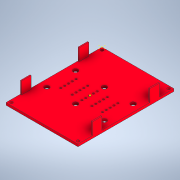
# Autodesk Inventor part: Base
Saved by Autodesk Inventor 2021 (Build 250183000, 183)
## iProperties
Created: 2025-01-23
Part Number: Base
Material: Generic
Document SubType Name: Modeling
Designer: User
Density: 1 g/cm^3
Appearance: Default
Author: User
Autodesk Inventor part; units mm, degrees
ref_plane "YZ Plane" through (0, 0, 0) normal (1, 0, 0) x (0, 1, 0)
ref_plane "XZ Plane" through (0, 0, 0) normal (0, 1, 0) x (-1, 0, 0)
ref_plane "XY Plane" through (0, 0, 0) normal (0, 0, 1) x (1, 0, 0)
sketch "Sketch1" plane through (0, 0, 0) normal (0, 1, 0) x (-1, 0, 0)
  line L0 (75, 0) -> (75, -100)
  line L1 (75, -100) -> (-75, -100)
  line L2 (-75, -100) -> (-75, 100)
  line L3 (-75, 100) -> (75, 100)
  line L4 (75, 100) -> (75, 0)
  line L5 (75, 100) -> (75, 70)
  line L6 (75, -100) -> (75, -70)
  line L7 (-75, -100) -> (-75, -70)
  line L8 (-75, 100) -> (-75, 70)
  line L9 (75, 70) -> (75, 50)
  line L10 (-75, 70) -> (-75, 50)
  line L11 (-75, -70) -> (-75, -50)
  line L12 (75, -70) -> (75, -50)
  line L13 (75, -70) -> (72.5, -70)
  line L14 (72.5, -70) -> (72.5, -50)
  line L15 (72.5, -50) -> (75, -50)
  line L16 (-75, -70) -> (-72.5, -70)
  line L17 (-72.5, -70) -> (-72.5, -50)
  line L18 (-72.5, -50) -> (-75, -50)
  line L19 (75, 70) -> (72.5, 70)
  line L20 (72.5, 70) -> (72.5, 50)
  line L21 (72.5, 50) -> (75, 50)
  line L22 (-75, 70) -> (-72.5, 70)
  line L23 (-72.5, 70) -> (-72.5, 50)
  line L24 (-72.5, 50) -> (-75, 50)
  line L25 (-75, -100) -> (-75, -97)
  line L26 (-75, -100) -> (-72, -100)
  circle A0 centre (-69.4679, -94.4422) radius 3
  circle A1 centre (69.3699, -94.4422) radius 3
  circle A2 centre (69.3699, 94.4217) radius 3
  circle A3 centre (-69.4679, 94.4217) radius 3
  line L27 (75, -50) -> (75, -35)
  line L28 (75, 50) -> (75, 35)
  line L29 (75, -35) -> (75, -25)
  line L30 (75, 35) -> (75, 25)
  line L31 (75, -25) -> (75, -21)
  line L32 (75, -21) -> (75, -17)
  line L33 (75, -17) -> (75, -13)
  line L34 (75, -13) -> (75, -9)
  line L35 (75, -9) -> (75, -5)
  line L36 (75, -5) -> (75, -1)
  line L37 (75, -1) -> (75, 3)
  line L38 (75, 3) -> (75, 7)
  line L39 (75, 7) -> (75, 11)
  line L40 (75, 11) -> (75, 15)
  line L41 (75, 15) -> (75, 19)
  line L42 (75, 19) -> (75, 23)
  circle A4 centre (60, 30) radius 5
  circle A5 centre (-60, 30) radius 5
  circle A6 centre (0, 30) radius 5
  line L43 (0, -35) -> (0, -30)
  circle A7 centre (0, -30) radius 5
  circle A8 centre (-60, -30) radius 5
  circle A9 centre (60, -30) radius 5
  circle A10 centre (0, -15) radius 2
  circle A11 centre (20, -15) radius 2
  circle A12 centre (44, -15) radius 2
  circle A13 centre (-21, -15) radius 2
  circle A14 centre (-43, -15) radius 2
  circle A15 centre (44, -7) radius 2
  circle A16 centre (20, -7) radius 2
  circle A17 centre (0, -7) radius 2
  circle A18 centre (-21, -7) radius 2
  circle A19 centre (-43, -7) radius 2
  circle A20 centre (44, 1) radius 2
  circle A21 centre (20, 1) radius 2
  circle A22 centre (0, 1) radius 2
  circle A23 centre (-21, 1) radius 2
  circle A24 centre (-43, 1) radius 2
  circle A25 centre (44, 9) radius 2
  circle A26 centre (20, 9) radius 2
  circle A27 centre (0, 9) radius 2
  circle A28 centre (-21, 9) radius 2
  circle A29 centre (-43, 9) radius 2
  circle A30 centre (44, 17) radius 2
  circle A31 centre (20, 17) radius 2
  circle A32 centre (0, 17) radius 2
  circle A33 centre (-21, 17) radius 2
  circle A34 centre (-43, 17) radius 2
  point P0 (0, 0)
  dimension "d3" = 150
  dimension "d4" = 200
  dimension "d6" = 30
  dimension "d7" = 30
  dimension "d8" = 30
  dimension "d9" = 30
  dimension "d10" = 20
  dimension "d11" = 20
  dimension "d12" = 20
  dimension "d13" = 20
  dimension "d14" = 2.5
  dimension "d15" = 2.5
  dimension "d16" = 2.5
  dimension "d17" = 2.5
  dimension "d20" = 6
  dimension "d23" = 6
  dimension "d26" = 6
  dimension "d28" = 6
  dimension "d30" = 15
  dimension "d31" = 15
  dimension "d32" = 10
  dimension "d33" = 10
  dimension "d34" = 4
  dimension "d35" = 4
  dimension "d47" = 10
  dimension "d49" = 10
  dimension "d50" = 10
  dimension "d51" = 5
  dimension "d52" = 10
  dimension "d55" = 10
  dimension "d56" = 10
  dimension "d58" = 4
  dimension "d59" = 4
  dimension "d60" = 4
  dimension "d61" = 4
  dimension "d62" = 4
  dimension "d63" = 4
  dimension "d64" = 4
  dimension "d65" = 4
  dimension "d66" = 4
  dimension "d67" = 4
  dimension "d68" = 4
  dimension "d69" = 4
  dimension "d70" = 4
  dimension "d71" = 4
  dimension "d72" = 4
  dimension "d73" = 4
  dimension "d74" = 4
  dimension "d75" = 4
  dimension "d76" = 4
  dimension "d77" = 4
  dimension "d78" = 4
  dimension "d79" = 4
  dimension "d80" = 4
  dimension "d81" = 4
  dimension "d82" = 4
  constraints: 84 end point, 35 centre point, 10 perpendicular, 6 point on line, 4 horizontal, 1 coincident, 1 vertical, 27 other
  measures "d3" distance of L1.start L1.end
  measures "d4" distance of L1.end L2.end
  measures "d6" distance of L3.end L5.end
  measures "d7" distance of L1.start L6.end
  measures "d8" distance of L1.end L7.end
  measures "d9" distance of L2.end L8.end
  measures "d10" distance of L5.end L9.end
  measures "d11" distance of L8.end L10.end
  measures "d12" distance of L7.end L11.end
  measures "d13" distance of L6.end L12.end
  measures "d14" distance of L6.end L13.end
  measures "d15" distance of L7.end L16.end
  measures "d16" distance of L5.end L19.end
  measures "d17" distance of L8.end L22.end
  measures "d20" diameter of A0
  measures "d23" diameter of A1
  measures "d26" diameter of A2
  measures "d28" diameter of A3
  measures "d30" distance of L12.end L27.end
  measures "d31" distance of L9.end L28.end
  measures "d32" distance of L27.end L29.end
  measures "d33" distance of L28.end L30.end
  measures "d34" distance of L29.end L31.end
  measures "d35" distance of L31.end L32.end
  measures "d47" diameter of A4
  measures "d49" diameter of A5
  measures "d50" diameter of A6
  measures "d51" distance of L43.start L43.end
  measures "d52" diameter of A7
  measures "d55" diameter of A8
  measures "d56" diameter of A9
  measures "d58" diameter of A10
  measures "d59" diameter of A11
  measures "d60" diameter of A12
  measures "d61" diameter of A13
  measures "d62" diameter of A14
  measures "d63" diameter of A15
  measures "d64" diameter of A16
  measures "d65" diameter of A17
  measures "d66" diameter of A18
  measures "d67" diameter of A19
  measures "d68" diameter of A20
  measures "d69" diameter of A21
  measures "d70" diameter of A22
  measures "d71" diameter of A23
  measures "d72" diameter of A24
  measures "d73" diameter of A25
  measures "d74" diameter of A26
  measures "d75" diameter of A27
  measures "d76" diameter of A28
  measures "d77" diameter of A29
  measures "d78" diameter of A30
  measures "d79" diameter of A31
  measures "d80" diameter of A32
  measures "d81" diameter of A33
  measures "d82" diameter of A34
extrude "Extrusion1" add sketch "Sketch1" along normal blind 5 contours L0 L15 L14 L13 L1 L2 L16 L17 L18 L24 L23 L22 L3 L4 L19 L20 L21
extrude "Extrusion2" add sketch "Sketch1" along normal blind 30 contours L2 L18 L17 L16
extrude "Extrusion3" add sketch "Sketch1" along normal blind 30 contours L0 L13 L14 L15
extrude "Extrusion4" add sketch "Sketch1" along normal blind 30 contours L21 L20 L19 L4
extrude "Extrusion5" add sketch "Sketch1" along normal blind 30 contours L22 L23 L24 L2
sketch "Sketch2" plane through (0, 5, 0) normal (0, 1, 0) x (1, 0, 0)
  point P0 (0, 0)
sketch "Sketch3" plane through (0, 5, 0) normal (0, 1, 0) x (1, 0, 0)
  point P0 (0, 0)
  point P1 (-75, 100)
body "Solid1"
